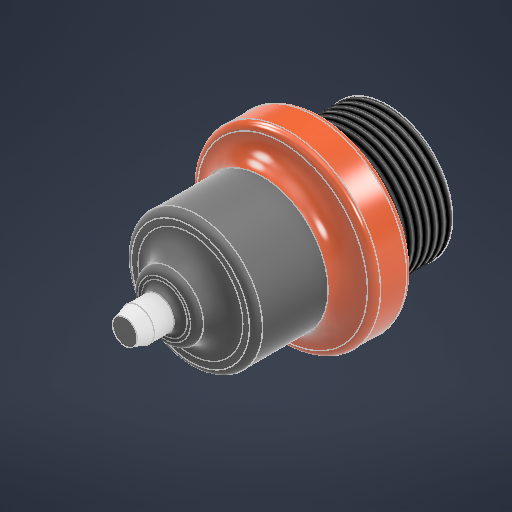
# Autodesk Inventor part: LOWER-NOZZLE
Saved by Autodesk Inventor 2025.3 (Build 293356030, 356C)
## iProperties
Created: 2025-08-28
Part Number: LOWER-NOZZLE
Material: PC/ABS Plastic
Document SubType Name: Modeling
Designer: lstk1ng
Density: 1.1 g/cm^3
Appearance: Smooth - Black
Mass: 379.049 g
Surface Area: 1384.9 cm^2
Volume: 344.59 cm^3
Author: lstk1ng
Autodesk Inventor part; units mm, degrees
ref_plane "YZ Plane" through (0, 0, 0) normal (1, 0, 0) x (0, 1, 0)
ref_plane "XZ Plane" through (0, 0, 0) normal (0, 1, 0) x (-1, 0, 0)
ref_plane "XY Plane" through (0, 0, 0) normal (0, 0, 1) x (1, 0, 0)
sketch "Sketch1" plane through (0, 0, 0) normal (0, 1, 0) x (-1, 0, 0)
  line L0 (50, 0) -> (50, 0) construction
  line L1 (0, -120) -> (0, 160) projected
  line L2 (50, -80) -> (0, -80)
  line L3 (50, -80) -> (50, -30)
  line L4 (50, -30) -> (65, -30)
  line L5 (70, -25) -> (70, -5)
  line L6 (65, 0) -> (65, 0)
  line L7 (50, 15) -> (50, 65)
  line L8 (45, 70) -> (40, 70)
  line L9 (25, 85) -> (25, 85)
  line L10 (20, 90) -> (17.5, 90)
  line L11 (12.5, 95) -> (12.5, 110)
  line L12 (9.5, 120) -> (0, 120)
  arc A0 (25, 85) -> (40, 70) centre (40, 85) ccw
  arc A1 (25, 85) -> (20, 90) centre (20, 85) ccw
  arc A2 (12.5, 95) -> (17.5, 90) centre (17.5, 95) ccw
  line L13 (9.5, 120) -> (12.5, 110)
  arc A3 (50, 65) -> (45, 70) centre (45, 65) ccw
  arc A4 (50, 15) -> (65, 0) centre (65, 15) ccw
  arc A5 (65, -30) -> (70, -25) centre (65, -25) ccw
  arc A6 (70, -5) -> (65, 0) centre (65, -5) ccw
  point P0 (0, 0)
  point P1 (35, 0)
  point P2 (70, -30)
  point P3 (70, 0)
  point P4 (50, 70)
  point P5 (25, 70)
  point P6 (25, 90)
  point P7 (12.5, 90)
  point P8 (12.5, 120)
  dimension "d1" = 80
  dimension "d28" = 50
  dimension "d29" = 20
  dimension "d30" = 70
  dimension "d31" = 25
  dimension "d32" = 20
  dimension "d33" = 12.5
  dimension "d34" = 30
  dimension "d35" = 15
  dimension "d36" = 5
  dimension "d37" = 3
  dimension "d38" = 10
  dimension "d39" = 5
  dimension "d44" = 15
  dimension "d45" = 5
  constraints: 26 end point, 20 point on line, 14 point on circle, 14 tangent, 7 centre point, 7 perpendicular, 3 horizontal, 2 equal radius, 2 vertical
  measures "d1" distance of L0.end L2.start
  measures "d28" distance of L2.start L3.end
  measures "d29" distance of L3.end point (70, -30)
  measures "d30" distance of L0.start point (50, 70)
  measures "d31" distance of point (50, 70) point (25, 70)
  measures "d32" distance of point (25, 70) point (25, 90)
  measures "d33" distance of point (25, 90) point (12.5, 90)
  measures "d34" distance of point (12.5, 90) point (12.5, 120)
  measures "d35" radius of A0
  measures "d36" radius of A1
  measures "d37" distance of L12.start point (12.5, 120)
  measures "d38" distance of L11.end point (12.5, 120)
  measures "d39" radius of A3
  measures "d44" radius of A4
  measures "d45" radius of A5
revolve "Revolution3" add sketch "Sketch1" angle 360 about axis through (0, 0, -10) along (0, 0, 1)
shell "Shell3" thickness 5 removed faces 1 at (11.7851, -15.9305, -80)
thread "Thread2" size "M100x6" class "6g" standard "ANSI Metric M Profile" length 50
body "Solid3"
